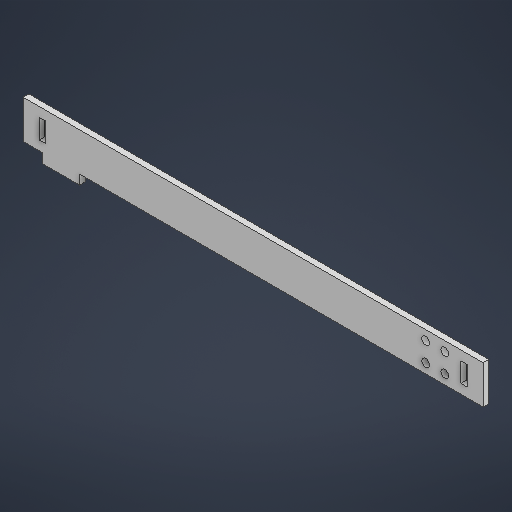
# Autodesk Inventor part: Middle_bar
Saved by Autodesk Inventor 2027 (Build 310192000, 192)
## iProperties
Created: 2026-05-09
Part Number: Middle_bar
Material: Generic
Document SubType Name: Modeling
Designer: alexy
Density: 1 g/cm^3
Appearance: Default
Author: alexy
Autodesk Inventor part; units mm, degrees
ref_plane "YZ Plane" through (0, 0, 0) normal (1, 0, 0) x (0, 1, 0)
ref_plane "XZ Plane" through (0, 0, 0) normal (0, 1, 0) x (-1, 0, 0)
ref_plane "XY Plane" through (0, 0, 0) normal (0, 0, 1) x (1, 0, 0)
sketch "Sketch1" plane through (0, 0, 0) normal (0, 0, 1) x (1, 0, 0)
  line L0 (0, 0) -> (240, 0)
  line L1 (240, 0) -> (240, 20)
  line L2 (240, 20) -> (0, 20)
  line L3 (0, 20) -> (0, 0)
  line L4 (0, 0) -> (22.0483, 0)
  line L5 (10, 0) -> (29.5, 0)
  line L6 (29.5, 0) -> (29.5, -5)
  line L7 (29.5, -5) -> (10, -5)
  line L8 (10, -5) -> (10, 0)
  line L9 (8.4, 15.1) -> (11.6, 15.1)
  line L10 (11.6, 15.1) -> (11.6, 4.9)
  line L11 (11.6, 4.9) -> (8.4, 4.9)
  line L12 (8.4, 4.9) -> (8.4, 15.1)
  line L13 (8.4, 15.1) -> (11.6, 4.9) construction
  line L14 (11.6, 15.1) -> (8.4, 4.9) construction
  line L15 (228.4, 15.1) -> (231.6, 15.1)
  line L16 (231.6, 15.1) -> (231.6, 4.9)
  line L17 (231.6, 4.9) -> (228.4, 4.9)
  line L18 (228.4, 4.9) -> (228.4, 15.1)
  line L19 (228.4, 15.1) -> (231.6, 4.9) construction
  line L20 (231.6, 15.1) -> (228.4, 4.9) construction
  circle A0 centre (220, 15) radius 2.05
  circle A1 centre (220, 5) radius 2.05
  circle A2 centre (210, 15) radius 2.05
  circle A3 centre (210, 5) radius 2.05
  point P0 (10, 10)
  point P1 (0, 10)
  point P2 (230, 10)
  dimension "d2" = 19.5
  dimension "d3" = 5
  dimension "d4" = 10
  dimension "d5" = 20
  dimension "d8" = 240
  dimension "d10" = 10.2
  dimension "d11" = 3.2
  dimension "d12" = 10
  dimension "d13" = 10.2
  dimension "d14" = 3.2
  dimension "d15" = 10
  dimension "d16" = 4.1
  dimension "d17" = 4.1
  dimension "d18" = 4.1
  dimension "d19" = 4.1
  dimension "d20" = 10
  dimension "d21" = 20
  dimension "d22" = 10
  dimension "d23" = 5
  constraints: 42 end point, 8 parallel, 5 horizontal, 5 midpoint, 4 centre point, 4 horizontal alignment, 4 perpendicular, 2 vertical alignment, 1 point on line
  measures "d2" distance of L6.end L7.end
  measures "d3" distance of L5.end L6.end
  measures "d4" distance of L0.start L5.start
  measures "d5" distance of L2.end L0.start
  measures "d8" distance of L1.end L2.end
  measures "d10" distance of L9.end L10.end
  measures "d11" distance of L10.end L11.end
  measures "d12" distance of point (0, 10) point (10, 10)
  measures "d13" distance of L16.start L16.end
  measures "d14" distance of L16.end L17.end
  measures "d15" distance from line of L1 point (230, 10)
  measures "d16" diameter of A0
  measures "d17" diameter of A1
  measures "d18" diameter of A2
  measures "d19" diameter of A3
  measures "d20" distance of A2.centre A0.centre
  measures "d21" distance from line of L1 A0.centre
  measures "d22" distance of A3.centre A2.centre
  measures "d23" distance from line of L2 A2.centre
extrude "Extrusion1" add sketch "Sketch1" along normal blind 3
body "Solid1"
